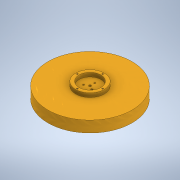
# Autodesk Inventor part: Wheel 2
Saved by Autodesk Inventor 2020 (Build 240168000, 168)
## iProperties
Created: 2020-02-18
Part Number: Wheel 2
Material: Brass, Soft Yellow, Welded
Document SubType Name: Modeling
Designer: user
Mass: 1655.85 g
Surface Area: 503.079 cm^2
Volume: 194.805 cm^3
Density: 8.5 g/cm^3
Appearance: Weld - Brass
Author: user
Autodesk Inventor part; units mm, degrees
ref_plane "YZ Plane" through (0, 0, 0) normal (1, 0, 0) x (0, 1, 0)
ref_plane "XZ Plane" through (0, 0, 0) normal (0, 1, 0) x (-1, 0, 0)
ref_plane "XY Plane" through (0, 0, 0) normal (0, 0, 1) x (1, 0, 0)
sketch "Sketch1" plane through (0, 0, 0) normal (0, 0, 1) x (1, 0, 0)
  line L0 (0, 20) -> (75, 20)
  line L1 (75, 20) -> (75, 0)
  line L2 (75, 0) -> (60, 0)
  line L3 (60, 0) -> (60, 14)
  line L4 (60, 14) -> (0, 14)
  line L5 (0, 14) -> (0, 20)
  line L6 (-15, 0) -> (90, 0) projected
  line L7 (0, -4) -> (0, 24) projected
  point P0 (0, 0)
  dimension "d2" = 14
  dimension "d3" = 20
  dimension "d5" = 150
  dimension "d6" = 120
  constraints: 12 end point, 4 perpendicular, 2 point on line, 1 horizontal, 1 parallel
  measures "d2" distance of L2.end L3.end
  measures "d3" distance of L0.end L1.end
  measures "d5" diameter of L0.end L5
  measures "d6" diameter of L2.end L5
revolve "Revolution1" add sketch "Sketch1" angle 360 about axis through (0, 14, 0) along (0, 1, 0) contours L0 L1 L2 L3 L4 L5
sketch "Sketch2" plane through (0, 20, 0) normal (0, 1, 0) x (1, 0, 0)
  circle A0 centre (0, 0) radius 75 projected
  circle A1 centre (0, 0) radius 2
  dimension "d7" = 4
  constraints: 1 centre point, 1 coincident
  measures "d7" diameter of A1
extrude "Extrusion1" cut sketch "Sketch2" against normal through all contours A1
sketch "Sketch3" plane through (0, 20, 0) normal (0, 1, 0) x (1, 0, 0)
  circle A0 centre (0, 0) radius 2 projected
  line L0 (0, 105) -> (0, -105) projected
  line L1 (-105, 0) -> (105, 0) projected
  point P0 (0, 8.5)
  point P1 (-7.3612, -4.25)
  point P2 (7.3612, -4.25)
  dimension "d10" = 8.5
  dimension "d13" = 360
  constraints: 1 point on line, 4 other
  measures "d10" distance of A0.centre point (0, 8.5)
hole "Hole1" at (0, 20, -8.5) at (-7.3612, 20, 4.25) at (7.3612, 20, 4.25) direction (0, -1, 0) diameter 3 end through all
sketch "Sketch4" plane through (0, 20, 0) normal (0, 1, 0) x (1, 0, 0)
  circle A0 centre (0, 0) radius 22.5
  circle A1 centre (0, 0) radius 25.5
  circle A2 centre (0, 0) radius 19.5
  dimension "d23" = 45
  dimension "d24" = 3
  dimension "d25" = 3
  constraints: 3 centre point, 1 coincident
  measures "d23" diameter of A0
  measures "d24" radial gap between concentric circles of A0 A1
  measures "d25" radial gap between concentric circles of A0 A2
extrude "Extrusion2" add sketch "Sketch4" along normal blind 7 contours A0 | A1
sketch "Sketch5" plane through (0, 27, 0) normal (0, 1, 0) x (1, 0, 0)
  circle A0 centre (0, 0) radius 22.5
  point P0 (-22.5, 0)
  point P1 (0, -22.5)
  point P2 (22.5, 0)
  point P3 (0, 22.5)
  dimension "d28" = 45
  constraints: 4 point on circle, 1 centre point, 1 coincident
  measures "d28" diameter of A0
hole "Hole2" at (-22.5, 27, 0) at (0, 27, 22.5) at (22.5, 27, 0) at (0, 27, -22.5) direction (0, -1, 0) diameter 2.459 depth 10 tip angle 118 thread size "M3x0.5" class "6H" standard "ANSI Metric M Profile"
body "Solid1"
